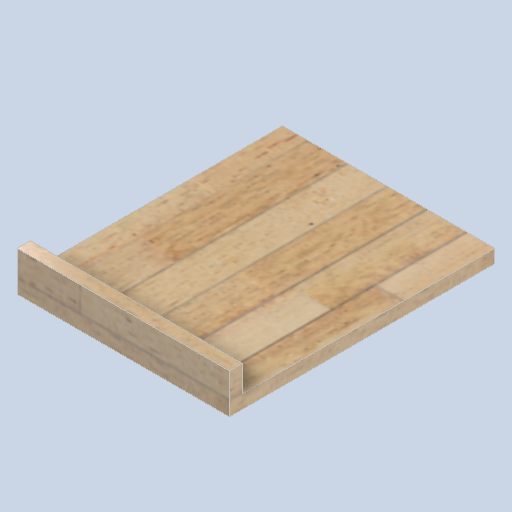
# Autodesk Inventor part: drawer
Saved by Autodesk Inventor 2022 (Build 260153000, 153)
## iProperties
Created: 2022-04-11
Part Number: drawer
Material: Wood (Maple)
Document SubType Name: Modeling
Designer: MacBook
Density: 0.67 g/cm^3
Appearance: Natural Maple - Glossy Dark Tint
Author: MacBook
Autodesk Inventor part; units mm, degrees
ref_plane "YZ Plane" through (0, 0, 0) normal (1, 0, 0) x (0, 1, 0)
ref_plane "XZ Plane" through (0, 0, 0) normal (0, 1, 0) x (-1, 0, 0)
ref_plane "XY Plane" through (0, 0, 0) normal (0, 0, 1) x (1, 0, 0)
sketch "Sketch1" plane through (0, 0, 0) normal (0, 1, 0) x (-1, 0, 0)
  line L0 (-152.4, -190.5) -> (152.4, -190.5)
  line L1 (152.4, -190.5) -> (152.4, 190.5)
  line L2 (152.4, 190.5) -> (-152.4, 190.5)
  line L3 (-152.4, 190.5) -> (-152.4, -190.5)
  line L4 (-152.4, -190.5) -> (152.4, 190.5) construction
  line L5 (152.4, -190.5) -> (-152.4, 190.5) construction
  point P0 (0, 0)
  dimension "d0" = 381
  dimension "d1" = 304.8
  constraints: 12 end point, 2 midpoint, 2 parallel, 1 horizontal, 1 perpendicular
  measures "d0" distance of L0.end L1.end
  measures "d1" distance between parallel lines of L3 L1
extrude "Extrusion1" add sketch "Sketch1" against normal blind 19.05
sketch "Sketch2" plane through (-152.4, 0, 190.5) normal (0, 0, 1) x (1, 0, 0)
  line L0 (0, 0) -> (304.8, 0)
  line L1 (304.8, 0) -> (304.8, 38.1)
  line L2 (304.8, 38.1) -> (0, 38.1)
  line L3 (0, 38.1) -> (0, 0)
  line L4 (304.8, 0) -> (304.8, -19.05) projected
  line L5 (0, 0) -> (0, -19.05) projected
  line L6 (304.8, -19.05) -> (0, -19.05) projected
  point P0 (152.4, 0)
  point P1 (304.8, -9.525)
  point P2 (304.8, 19.05)
  dimension "d4" = 0
  dimension "d5" = 38.1
  dimension "d6" = 0
  dimension "d7" = 19.05
  constraints: 8 end point, 2 midpoint, 2 parallel, 1 horizontal, 1 perpendicular
  measures "d4" horizontal distance of point (304.8, -9.525) point (304.8, 19.05)
  measures "d5" distance between parallel lines of L0 L2
  measures "d6" distance between parallel lines of L5 L3
  measures "d7" distance between parallel lines of L6 L0
extrude "Extrusion2" add sketch "Sketch2" against normal blind 19.05 contours L3 L2 L1 L0
body "Solid1"
